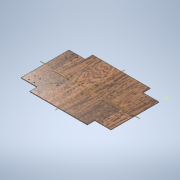
# Autodesk Inventor part: base
Saved by Autodesk Inventor 2022 (Build 260153000, 153)
## iProperties
Created: 2023-03-09
Part Number: base
Material: 一般
Document SubType Name: Modeling
Designer: JOU
Density: 1 g/cm^3
Appearance: 預設
Author: JOU
Autodesk Inventor part; units mm, degrees
ref_plane "YZ Plane" through (0, 0, 0) normal (1, 0, 0) x (0, 1, 0)
ref_plane "XZ Plane" through (0, 0, 0) normal (0, 1, 0) x (-1, 0, 0)
ref_plane "XY Plane" through (0, 0, 0) normal (0, 0, 1) x (1, 0, 0)
sketch "草圖1" plane through (0, 0, 0) normal (0, 1, 0) x (-1, 0, 0)
  point P0 (0, 0)
sketch "草圖2" plane through (0, 0, 0) normal (0, 1, 0) x (-1, 0, 0)
  line L0 (0, 0) -> (300, 0)
  line L1 (300, 0) -> (300, 210)
  line L2 (300, 210) -> (0, 210)
  line L3 (0, 210) -> (0, 0)
  dimension "d0" = 210
  dimension "d1" = 300
  constraints: 8 end point, 2 parallel, 1 horizontal, 1 perpendicular
  measures "d0" distance of L0.end L1.end
  measures "d1" distance of L1.end L2.end
extrude "擠出1" add sketch "草圖2" along normal blind 2
sketch "草圖4" plane through (0, 2, 0) normal (0, 1, 0) x (1, 0, 0)
  line L0 (-300, 0) -> (-300, -210) projected
  line L1 (-300, -210) -> (-246, -210)
  line L2 (-246, -210) -> (-246, -185)
  line L3 (-246, -185) -> (-300, -185)
  line L4 (-300, -185) -> (-300, -210)
  line L5 (-300, 0) -> (-246, 0)
  line L6 (-246, 0) -> (-246, -25)
  line L7 (-246, -25) -> (-300, -25)
  line L8 (-300, -25) -> (-300, 0)
  line L9 (0, 0) -> (-300, 0) projected
  line L10 (0, 0) -> (-54, 0)
  line L11 (-54, 0) -> (-54, -25)
  line L12 (-54, -25) -> (0, -25)
  line L13 (0, -25) -> (0, 0)
  line L14 (0, -210) -> (0, 0) projected
  line L15 (0, -210) -> (-54, -210)
  line L16 (-54, -210) -> (-54, -185)
  line L17 (-54, -185) -> (0, -185)
  line L18 (0, -185) -> (0, -210)
  dimension "d9" = 54
  dimension "d10" = 25
  constraints: 32 end point, 8 parallel, 6 equal length, 4 horizontal, 4 perpendicular
  measures "d9" distance of L2.end L3.end
  measures "d10" distance of L1.end L2.end
extrude "擠出3" cut sketch "草圖4" against normal up to surface (2 mm away)
sketch "草圖5" plane through (0, 2, 0) normal (0, 1, 0) x (1, 0, 0)
  circle A0 centre (-281.5, -33) radius 1.5
  circle A1 centre (-264.5, -33) radius 1.5
  circle A2 centre (-281.5, -53) radius 1.5
  circle A3 centre (-264.5, -53) radius 1.5
  line L0 (-281.5, -33) -> (-264.5, -33)
  line L1 (-273, -33) -> (-273, -53.0368)
  line L2 (-300, -25) -> (-300, -185) projected
  line L3 (-246, -25) -> (-300, -25) projected
  point P0 (0, 0)
  dimension "d13" = 3
  dimension "d14" = 17
  dimension "d16" = 20
  dimension "d17" = 27
  dimension "d20" = 8
  constraints: 4 centre point, 4 end point, 3 equal radius, 2 horizontal alignment, 2 vertical alignment, 1 horizontal, 1 midpoint, 1 vertical
  measures "d13" diameter of A0
  measures "d14" distance of L0.end L0.start
  measures "d16" distance of A2.centre L0.start
  measures "d17" distance between parallel lines of L2 L1
  measures "d20" distance between parallel lines of L3 L0
extrude "擠出4" cut sketch "草圖5" against normal up to surface (2 mm away)
ref_plane "工作平面2" through (-150, 0, 25) normal (-1, 0, 0) x (0, 0, 1)
ref_plane "工作平面1" through (-54, 0, 105) normal (0, 0, -1) x (-1, 0, 0)
mirror "鏡射1" about plane through (-54, 0, 105) normal (0, 0, -1) of "擠出4"
mirror "鏡射2" about plane through (-150, 0, 25) normal (-1, 0, 0) of "擠出4", "鏡射1"
sketch "草圖6" plane through (0, 2, 0) normal (0, 1, 0) x (1, 0, 0)
  line L0 (-150, -252) -> (-150, 42) projected
  line L1 (-530.8667, -105) -> (88.4778, -105) projected
  circle A0 centre (-150, -81) radius 2
  circle A1 centre (-97.5, -94.5) radius 2
  circle A2 centre (-97.5, -123.5) radius 2
  circle A3 centre (-150, -129) radius 2
  circle A4 centre (-150, -81) radius 2
  circle A5 centre (-97.5, -94.5) radius 2
  circle A6 centre (-97.5, -123.5) radius 2
  circle A7 centre (-150, -129) radius 2
  line L2 (-150, -81) -> (-150, -129)
  line L3 (-150, -105) -> (-130.1449, -105)
  circle A8 centre (-217, -62.5) radius 1.5
  circle A9 centre (-180, -62.5) radius 1.5
  circle A10 centre (-180, -99.5) radius 1.5
  circle A11 centre (-217, -99.5) radius 1.5
  line L4 (-180, -62.5) -> (-180, -99.5)
  line L5 (-180, -81) -> (-200.7976, -81)
  line L6 (-150, -81) -> (-180, -81)
  line L7 (-150, -129) -> (-180, -129)
  circle A12 centre (-217, -110.5) radius 1.5
  circle A13 centre (-180, -110.5) radius 1.5
  circle A14 centre (-180, -147.5) radius 1.5
  circle A15 centre (-217, -147.5) radius 1.5
  line L8 (-180, -110.5) -> (-180, -147.5)
  line L9 (-180, -129) -> (-200.7976, -129)
  circle A16 centre (-97.5, -115.5) radius 2
  circle A17 centre (-97.5, -86.5) radius 2
  circle A18 centre (-97.5, -115.5) radius 2
  circle A19 centre (-97.5, -86.5) radius 2
  point P0 (0, 0)
  dimension "d23" = 30
  dimension "d24" = 30
  constraints: 20 centre point, 16 end point, 6 horizontal, 4 midpoint, 4 symmetric about line, 4 vertical, 1 point on line, 32 other
  measures "d23" distance of L2.start L6.end
  measures "d24" distance of L2.end L7.end
extrude "擠出5" cut sketch "草圖6" against normal up to surface (2 mm away) contours A3 L7 L0 | L0 A3 | L7 A3 L0 | A0 L6 L0 | L0 A0 | L6 A0 L0 | A8 | A9 | A10 | A11 | A12 | A13 | A14 | A15 | A16 | A17
equation "\"d0\" = W_"
equation "\"d1\" = L_"
equation "\"d2\" = h_"
equation "\"d9\" = wheel_d"
equation "\"d10\" = wheel_w"
equation "\"d13\" = screw_hole"
equation "\"W_\" = 210"
equation "\"L_\" = 300"
equation "\"h_\" = 2"
equation "\"wheel_d\" = 54"
equation "\"wheel_w\" = 25"
equation "\"screw_hole\" = 3"
